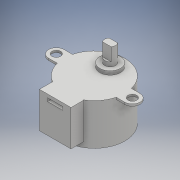
# Autodesk Inventor part: 28BYJ-48
Saved by Autodesk Inventor 2018.3 (Build 223284000, 284)
## iProperties
Created: 2019-02-23
Part Number: 28BYJ-48
Material: 一般
Document SubType Name: Modeling
Designer: shun2
Density: 1 g/cm^3
Appearance: 既定
Author: shun2
Autodesk Inventor part; units mm, degrees
ref_plane "YZ Plane" through (0, 0, 0) normal (1, 0, 0) x (0, 1, 0)
ref_plane "XZ Plane" through (0, 0, 0) normal (0, 1, 0) x (-1, 0, 0)
ref_plane "XY Plane" through (0, 0, 0) normal (0, 0, 1) x (1, 0, 0)
sketch "スケッチ1" plane through (0, 0, 0) normal (0, 0, 1) x (1, 0, 0)
  circle A0 centre (0, 0) radius 14
  dimension "d0" = 28
  constraints: 1 centre point, 1 coincident
  measures "d0" diameter of A0
extrude "押し出し1" add sketch "スケッチ1" along normal blind 19
sketch "スケッチ2" plane through (0, 0, 19) normal (0, 0, 1) x (1, 0, 0)
  circle A0 centre (0, 0) radius 14 projected
  arc A1 (-17.5, 3.5) -> (-17.5, -3.5) centre (-17.5, 0) ccw
  arc A2 (17.5, -3.5) -> (17.5, 3.5) centre (17.5, 0) ccw
  line L0 (-17.5, 3.5) -> (-13.5554, 3.5)
  line L1 (-17.5, -3.5) -> (-13.5554, -3.5)
  line L2 (13.5554, 3.5) -> (17.5, 3.5)
  line L3 (13.5554, -3.5) -> (17.5, -3.5)
  circle A3 centre (-17.5, 0) radius 2
  circle A4 centre (17.5, 0) radius 2
  dimension "d5" = 7
  dimension "d6" = 7
  dimension "d7" = 4
  dimension "d8" = 4
  constraints: 8 end point, 8 point on circle, 4 centre point, 4 point on line, 2 coincident, 1 horizontal, 1 parallel
  measures "d5" diameter of A1
  measures "d6" diameter of A2
  measures "d7" diameter of A3
  measures "d8" diameter of A4
extrude "押し出し2" add sketch "スケッチ2" against normal blind 0.9 contours A0 L2 A2 L3 | A0 L1 A1 L0
sketch "スケッチ3" plane through (0, 0, 19) normal (0, 0, 1) x (1, 0, 0)
  line L0 (-7.25, -14) -> (-7.25, -18)
  line L1 (-7.25, -18) -> (7.25, -18)
  line L2 (7.25, -18) -> (7.25, -14)
  line L3 (-7.25, -14) -> (-7.25, -12.0918)
  line L4 (7.25, -14) -> (7.25, -12.0918)
  circle A0 centre (-17.5, 0) radius 2 projected
  circle A1 centre (17.5, 0) radius 2 projected
  arc A2 (13.5554, 3.5) -> (-13.5554, 3.5) centre (0, 0) ccw projected
  line L5 (-13.5554, 3.5) -> (-17.5, 3.5) projected
  arc A3 (-17.5, 3.5) -> (-17.5, -3.5) centre (-17.5, 0) ccw projected
  line L6 (-17.5, -3.5) -> (-13.5554, -3.5) projected
  arc A4 (-13.5554, -3.5) -> (13.5554, -3.5) centre (0, 0) ccw projected
  line L7 (13.5554, -3.5) -> (17.5, -3.5) projected
  arc A5 (17.5, -3.5) -> (17.5, 3.5) centre (17.5, 0) ccw projected
  line L8 (17.5, 3.5) -> (13.5554, 3.5) projected
  line L9 (7.25, -12.0918) -> (-7.25, -12.0918)
  line L10 (-7.25, -12.0918) -> (-7.25, -18)
  line L11 (-7.25, -18) -> (7.25, -18)
  line L12 (7.25, -18) -> (7.25, -12.0918)
  constraints: 18 end point, 3 parallel, 2 vertical, 1 horizontal, 1 perpendicular
extrude "押し出し3" add sketch "スケッチ3" against normal blind 16.5 contours L3 L9 A4 L4 L2 L1 L0 | L9 A4
sketch "スケッチ4" plane through (0, 0, 19) normal (0, 0, 1) x (1, 0, 0)
  arc A0 (7.056, -12.0918) -> (13.5554, -3.5) centre (0, 0) ccw projected
  line L0 (13.5554, -3.5) -> (17.5, -3.5) projected
  arc A1 (17.5, -3.5) -> (17.5, 3.5) centre (17.5, 0) ccw projected
  line L1 (17.5, 3.5) -> (13.5554, 3.5) projected
  arc A2 (13.5554, 3.5) -> (-13.5554, 3.5) centre (0, 0) ccw projected
  line L2 (-13.5554, 3.5) -> (-17.5, 3.5) projected
  arc A3 (-17.5, 3.5) -> (-17.5, -3.5) centre (-17.5, 0) ccw projected
  line L3 (-17.5, -3.5) -> (-13.5554, -3.5) projected
  arc A4 (-13.5554, -3.5) -> (-7.056, -12.0918) centre (0, 0) ccw projected
  line L4 (-7.25, -12.0918) -> (-7.056, -12.0918) projected
  line L5 (-7.25, -18) -> (-7.25, -12.0918) projected
  line L6 (7.25, -18) -> (-7.25, -18) projected
  line L7 (7.25, -12.0918) -> (7.25, -18) projected
  line L8 (7.056, -12.0918) -> (7.25, -12.0918) projected
  circle A5 centre (-17.5, 0) radius 2 projected
  circle A6 centre (17.5, 0) radius 2 projected
  circle A7 centre (0, 7.25) radius 4.75
  dimension "d15" = 9.5
  constraints: 1 centre point
  measures "d15" diameter of A7
extrude "押し出し4" add sketch "スケッチ4" along normal blind 1.7 contours A7
sketch "スケッチ5" plane through (0, 7.25, 20.7) normal (0, 0, 1) x (1, 0, 0)
  circle A0 centre (0, 0) radius 2.5
  point P0 (0, -7.25)
  dimension "d18" = 5
  constraints: 1 centre point
  measures "d18" diameter of A0
extrude "押し出し5" add sketch "スケッチ5" along normal blind 8
sketch "スケッチ6" plane through (0, 7.25, 28.7) normal (0, 0, 1) x (1, 0, 0)
  circle A0 centre (0, 0) radius 2.5 projected
  line L0 (2, 1.5) -> (-2, 1.5)
  line L1 (-2, -1.5) -> (2, -1.5)
  circle A1 centre (0, 0) radius 2.5
  point P0 (0, -7.25)
  dimension "d23" = 5
  constraints: 4 end point, 4 point on circle, 1 centre point, 1 coincident, 1 horizontal, 1 parallel
  measures "d23" diameter of A1
extrude "押し出し6" cut sketch "スケッチ6" against normal blind 6 contours L0 A0 | A0 L1
sketch "スケッチ7" plane through (-7.25, -18, 19) normal (0, -1, 0) x (1, 0, 0)
  line L0 (3.75, -1.5) -> (10.75, -1.5)
  line L1 (10.75, -1.5) -> (10.75, -3)
  line L2 (10.75, -3) -> (3.75, -3)
  line L3 (3.75, -3) -> (3.75, -1.5)
  point P0 (7.25, -19)
  dimension "d26" = 7
  dimension "d27" = 1.5
  constraints: 8 end point, 2 parallel, 1 horizontal, 1 perpendicular
  measures "d26" distance of L1.end L2.end
  measures "d27" distance of L0.end L1.end
extrude "押し出し7" cut sketch "スケッチ7" against normal blind 5
